Autodesk Inventor part; units mm, degrees
(part 2 of 2)
  line L990 (56.4, 473.8891) -> (43.8, 481.1637)
  line L991 (43.8, 481.1637) -> (43.8, 495.7129)
  line L992 (43.8, 495.7129) -> (56.4, 502.9876)
  line L993 (42.3, 527.4095) -> (54.9, 520.1349)
  line L994 (54.9, 520.1349) -> (54.9, 505.5856)
  line L995 (54.9, 505.5856) -> (42.3, 498.311)
  line L996 (42.3, 498.311) -> (29.7, 505.5856)
  line L997 (29.7, 505.5856) -> (29.7, 520.1349)
  line L998 (29.7, 520.1349) -> (42.3, 527.4095)
  line L999 (28.2, 551.8314) -> (40.8, 544.5568)
  line L1000 (40.8, 544.5568) -> (40.8, 530.0075)
  line L1001 (40.8, 530.0075) -> (28.2, 522.7329)
  line L1002 (28.2, 522.7329) -> (15.6, 530.0075)
  line L1003 (15.6, 530.0075) -> (15.6, 544.5568)
  line L1004 (15.6, 544.5568) -> (28.2, 551.8314)
  line L1005 (14.1, 576.2533) -> (26.7, 568.9787)
  line L1006 (26.7, 568.9787) -> (26.7, 554.4295)
  line L1007 (26.7, 554.4295) -> (14.1, 547.1549)
  line L1008 (14.1, 547.1549) -> (1.5, 554.4295)
  line L1009 (1.5, 554.4295) -> (1.5, 568.9787)
  line L1010 (1.5, 568.9787) -> (14.1, 576.2533)
  line L1011 (0, 600.6752) -> (12.6, 593.4006)
  line L1012 (12.6, 593.4006) -> (12.6, 578.8514)
  line L1013 (12.6, 578.8514) -> (0, 571.5768)
  line L1014 (0, 571.5768) -> (-12.6, 578.8514)
  line L1015 (-12.6, 578.8514) -> (-12.6, 593.4006)
  line L1016 (-12.6, 593.4006) -> (0, 600.6752)
  line L1017 (75, 218.063) -> (-75, 218.063)
  line L1018 (-75, 218.063) -> (-75, 368.063)
  line L1019 (-75, 368.063) -> (75, 368.063)
  line L1020 (75, 368.063) -> (75, 218.063)
  line L1021 (75, 218.063) -> (-75, 368.063) construction
  line L1022 (-75, 218.063) -> (75, 368.063) construction
  point P0 (-14.1, 24.4219)
  point P1 (-20.4, 35.3338)
  point P2 (-7.6023, 35.6763)
  point P3 (-28.2, 48.8438)
  point P4 (-34.5, 59.7558)
  point P5 (-21.7023, 60.0982)
  point P6 (-42.3, 73.2657)
  point P7 (-48.6, 84.1777)
  point P8 (-35.8023, 84.5201)
  point P9 (-56.4, 97.6877)
  point P10 (-62.7, 108.5996)
  point P11 (-49.9023, 108.942)
  point P12 (-70.5, 122.1096)
  point P13 (-76.8, 133.0215)
  point P14 (-64.0023, 133.364)
  point P15 (-84.6, 146.5315)
  point P16 (-90.9, 157.4434)
  point P17 (-78.1023, 157.7859)
  point P18 (-98.7, 170.9534)
  point P19 (-105, 181.8653)
  point P20 (-92.2023, 182.2078)
  point P21 (-112.8, 195.3753)
  point P22 (-119.1, 206.2873)
  point P23 (-106.3023, 206.6297)
  point P24 (-126.9, 219.7972)
  point P25 (-133.2, 230.7092)
  point P26 (-120.4023, 231.0516)
  point P27 (-141, 244.2192)
  point P28 (-147.3, 255.1311)
  point P29 (-134.5023, 255.4735)
  point P30 (-155.1, 268.6411)
  point P31 (-161.4, 279.553)
  point P32 (-148.6023, 279.8955)
  point P33 (-169.2, 293.063)
  point P34 (-175.5, 303.9749)
  point P35 (-162.7023, 304.3174)
  point P36 (14.1, 24.4219)
  point P37 (7.8, 35.3338)
  point P38 (20.5977, 35.6763)
  point P39 (0, 48.8438)
  point P40 (-6.3, 59.7558)
  point P41 (6.4977, 60.0982)
  point P42 (-14.1, 73.2657)
  point P43 (-20.4, 84.1777)
  point P44 (-7.6023, 84.5201)
  point P45 (-28.2, 97.6877)
  point P46 (-34.5, 108.5996)
  point P47 (-21.7023, 108.942)
  point P48 (-42.3, 122.1096)
  point P49 (-48.6, 133.0215)
  point P50 (-35.8023, 133.364)
  point P51 (-56.4, 146.5315)
  point P52 (-62.7, 157.4434)
  point P53 (-49.9023, 157.7859)
  point P54 (-70.5, 170.9534)
  point P55 (-76.8, 181.8653)
  point P56 (-64.0023, 182.2078)
  point P57 (-84.6, 195.3753)
  point P58 (-90.9, 206.2873)
  point P59 (-78.1023, 206.6297)
  point P60 (-98.7, 219.7972)
  point P61 (-105, 230.7092)
  point P62 (-92.2023, 231.0516)
  point P63 (-112.8, 244.2192)
  point P64 (-119.1, 255.1311)
  point P65 (-106.3023, 255.4735)
  point P66 (-126.9, 268.6411)
  point P67 (-133.2, 279.553)
  point P68 (-120.4023, 279.8955)
  point P69 (-141, 293.063)
  point P70 (-147.3, 303.9749)
  point P71 (-134.5023, 304.3174)
  point P72 (-155.1, 317.4849)
  point P73 (-161.4, 328.3968)
  point P74 (-148.6023, 328.7393)
  point P75 (28.2, 48.8438)
  point P76 (21.9, 59.7558)
  point P77 (34.6977, 60.0982)
  point P78 (14.1, 73.2657)
  point P79 (7.8, 84.1777)
  point P80 (20.5977, 84.5201)
  point P81 (0, 97.6877)
  point P82 (-6.3, 108.5996)
  point P83 (6.4977, 108.942)
  point P84 (-14.1, 122.1096)
  point P85 (-20.4, 133.0215)
  point P86 (-7.6023, 133.364)
  point P87 (-28.2, 146.5315)
  point P88 (-34.5, 157.4434)
  point P89 (-21.7023, 157.7859)
  point P90 (-42.3, 170.9534)
  point P91 (-48.6, 181.8653)
  point P92 (-35.8023, 182.2078)
  point P93 (-56.4, 195.3753)
  point P94 (-62.7, 206.2873)
  point P95 (-49.9023, 206.6297)
  point P96 (-70.5, 219.7972)
  point P97 (-76.8, 230.7092)
  point P98 (-64.0023, 231.0516)
  point P99 (-84.6, 244.2192)
  point P100 (-90.9, 255.1311)
  point P101 (-78.1023, 255.4735)
  point P102 (-98.7, 268.6411)
  point P103 (-105, 279.553)
  point P104 (-92.2023, 279.8955)
  point P105 (-112.8, 293.063)
  point P106 (-119.1, 303.9749)
  point P107 (-106.3023, 304.3174)
  point P108 (-126.9, 317.4849)
  point P109 (-133.2, 328.3968)
  point P110 (-120.4023, 328.7393)
  point P111 (-141, 341.9068)
  point P112 (-147.3, 352.8187)
  point P113 (-134.5023, 353.1612)
  point P114 (42.3, 73.2657)
  point P115 (36, 84.1777)
  point P116 (48.7977, 84.5201)
  point P117 (28.2, 97.6877)
  point P118 (21.9, 108.5996)
  point P119 (34.6977, 108.942)
  point P120 (14.1, 122.1096)
  point P121 (7.8, 133.0215)
  point P122 (20.5977, 133.364)
  point P123 (0, 146.5315)
  point P124 (-6.3, 157.4434)
  point P125 (6.4977, 157.7859)
  point P126 (-14.1, 170.9534)
  point P127 (-20.4, 181.8653)
  point P128 (-7.6023, 182.2078)
  point P129 (-28.2, 195.3753)
  point P130 (-34.5, 206.2873)
  point P131 (-21.7023, 206.6297)
  point P132 (-42.3, 219.7972)
  point P133 (-48.6, 230.7092)
  point P134 (-35.8023, 231.0516)
  point P135 (-56.4, 244.2192)
  point P136 (-62.7, 255.1311)
  point P137 (-49.9023, 255.4735)
  point P138 (-70.5, 268.6411)
  point P139 (-76.8, 279.553)
  point P140 (-64.0023, 279.8955)
  point P141 (-84.6, 293.063)
  point P142 (-90.9, 303.9749)
  point P143 (-78.1023, 304.3174)
  point P144 (-98.7, 317.4849)
  point P145 (-105, 328.3968)
  point P146 (-92.2023, 328.7393)
  point P147 (-112.8, 341.9068)
  point P148 (-119.1, 352.8187)
  point P149 (-106.3023, 353.1612)
  point P150 (-126.9, 366.3287)
  point P151 (-133.2, 377.2407)
  point P152 (-120.4023, 377.5831)
  point P153 (56.4, 97.6877)
  point P154 (50.1, 108.5996)
  point P155 (62.8977, 108.942)
  point P156 (42.3, 122.1096)
  point P157 (36, 133.0215)
  point P158 (48.7977, 133.364)
  point P159 (28.2, 146.5315)
  point P160 (21.9, 157.4434)
  point P161 (34.6977, 157.7859)
  point P162 (14.1, 170.9534)
  point P163 (7.8, 181.8653)
  point P164 (20.5977, 182.2078)
  point P165 (0, 195.3753)
  point P166 (-6.3, 206.2873)
  point P167 (6.4977, 206.6297)
  point P168 (-14.1, 219.7972)
  point P169 (-20.4, 230.7092)
  point P170 (-7.6023, 231.0516)
  point P171 (-28.2, 244.2192)
  point P172 (-34.5, 255.1311)
  point P173 (-21.7023, 255.4735)
  point P174 (-42.3, 268.6411)
  point P175 (-48.6, 279.553)
  point P176 (-35.8023, 279.8955)
  point P177 (-56.4, 293.063)
  point P178 (-62.7, 303.9749)
  point P179 (-49.9023, 304.3174)
  point P180 (-70.5, 317.4849)
  point P181 (-76.8, 328.3968)
  point P182 (-64.0023, 328.7393)
  point P183 (-84.6, 341.9068)
  point P184 (-90.9, 352.8187)
  point P185 (-78.1023, 353.1612)
  point P186 (-98.7, 366.3287)
  point P187 (-105, 377.2407)
  point P188 (-92.2023, 377.5831)
  point P189 (-112.8, 390.7507)
  point P190 (-119.1, 401.6626)
  point P191 (-106.3023, 402.005)
  point P192 (70.5, 122.1096)
  point P193 (64.2, 133.0215)
  point P194 (76.9977, 133.364)
  point P195 (56.4, 146.5315)
  point P196 (50.1, 157.4434)
  point P197 (62.8977, 157.7859)
  point P198 (42.3, 170.9534)
  point P199 (36, 181.8653)
  dimension "d0" = 14.5492
  dimension "d3" = 28.2
  dimension "d6" = 28.2
  dimension "d40" = 150
  dimension "d41" = 150
  constraints: 2046 end point, 171 midpoint, 3 perpendicular, 2 parallel, 1 coincident, 1 horizontal, 1 vertical, 2535 other
  measures "d0" distance of L0.start L0.end
  measures "d3" distance of L0.end L9.start
  measures "d6" distance of L0.end L81.start
  measures "d40" distance of L1018.end L1019.end
  measures "d41" distance of L1017.end L1018.end
extrude "Extrusion_HoneyComb" add sketch "Sketch1" along normal blind 3 contours L206 L1018 L209 L208 L207 L288 L287 L286 L285 L290 L293 L292 L291 L372 L371 L370 L369 L374 L377 L376 L375 L456 L455 L454 L1019 L529 L528 L527 L526 L601 L600 L599 L598 L673 L672 L671 L670 L745 L744 L743 L742 L817 L816 L815 L1020 L812 L811 L810 L729 L734 L733 L732 L731 L728 L727 L726 L645 L650 L649 L648 L647 L644 L643 L642 L561 L566 L565 L1017 L490 L489 L494 L493 L418 L417 L422 L421 L346 L345 L350 L349 L274 L273 L278 L277 L202 L201 | L201 L202 L1017 L1018 L206 | L1018 L207 L208 L209 | L277 L278 L273 L274 L1017 | L1018 L290 L285 L286 L287 L288 | L349 L350 L345 L346 L1017 | L1018 L291 L292 L293 | L421 L422 L417 L418 L1017 | L1018 L374 L369 L370 L371 L372 | L493 L494 L489 L490 L1017 | L1018 L375 L376 L377 | L565 L566 L561 L1020 L1017 | L1018 L1019 L454 L455 L456 | L642 L643 L644 L1020 | L1019 L526 L527 L528 L529 | L647 L648 L649 L650 L645 L1020 | L1019 L598 L599 L600 L601 | L726 L727 L728 L1020 | L1019 L670 L671 L672 L673 | L731 L732 L733 L734 L729 L1020 | L1019 L742 L743 L744 L745 | L810 L811 L812 L1020 | L1019 L1020 L815 L816 L817
sketch "Sketch2" plane through (0, 0, 0) normal (0, 0, -1) x (-1, 0, 0)
  line L0 (-75, 368.063) -> (-75, 218.063) projected
  line L1 (-75, 368.063) -> (-72, 368.063)
  line L2 (-72, 368.063) -> (-72, 330.563)
  line L3 (-72, 330.563) -> (-75, 330.563)
  line L4 (-75, 330.563) -> (-75, 368.063)
  line L5 (-75, 330.563) -> (-72, 330.563)
  line L6 (-72, 330.563) -> (-72, 293.063)
  line L7 (-72, 293.063) -> (-75, 293.063)
  line L8 (-75, 293.063) -> (-75, 330.563)
  line L9 (-75, 293.063) -> (-72, 293.063)
  line L10 (-72, 293.063) -> (-72, 255.563)
  line L11 (-72, 255.563) -> (-75, 255.563)
  line L12 (-75, 255.563) -> (-75, 293.063)
  line L13 (75, 218.063) -> (-75, 218.063) projected
  line L14 (-75, 255.563) -> (-72, 255.563)
  line L15 (-72, 255.563) -> (-72, 218.063)
  line L16 (-72, 218.063) -> (-75, 218.063)
  line L17 (-75, 218.063) -> (-75, 255.563)
  line L18 (-75, 218.063) -> (-37.5, 218.063)
  line L19 (-37.5, 218.063) -> (-37.5, 221.063)
  line L20 (-37.5, 221.063) -> (-75, 221.063)
  line L21 (-75, 221.063) -> (-75, 218.063)
  line L22 (-37.5, 218.063) -> (0, 218.063)
  line L23 (0, 218.063) -> (0, 221.063)
  line L24 (0, 221.063) -> (-37.5, 221.063)
  line L25 (-37.5, 221.063) -> (-37.5, 218.063)
  line L26 (0, 218.063) -> (37.5, 218.063)
  line L27 (37.5, 218.063) -> (37.5, 221.063)
  line L28 (37.5, 221.063) -> (0, 221.063)
  line L29 (0, 221.063) -> (0, 218.063)
  line L30 (75, 368.063) -> (75, 218.063) projected
  line L31 (37.5, 218.063) -> (75, 218.063)
  line L32 (75, 218.063) -> (75, 221.063)
  line L33 (75, 221.063) -> (37.5, 221.063)
  line L34 (37.5, 221.063) -> (37.5, 218.063)
  line L35 (75, 218.063) -> (72, 218.063)
  line L36 (72, 218.063) -> (72, 255.563)
  line L37 (72, 255.563) -> (75, 255.563)
  line L38 (75, 255.563) -> (75, 218.063)
  line L39 (75, 255.563) -> (72, 255.563)
  line L40 (72, 255.563) -> (72, 293.063)
  line L41 (72, 293.063) -> (75, 293.063)
  line L42 (75, 293.063) -> (75, 255.563)
  line L43 (75, 293.063) -> (72, 293.063)
  line L44 (72, 293.063) -> (72, 330.563)
  line L45 (72, 330.563) -> (75, 330.563)
  line L46 (75, 330.563) -> (75, 293.063)
  line L47 (-75, 368.063) -> (75, 368.063) projected
  line L48 (75, 330.563) -> (72, 330.563)
  line L49 (72, 330.563) -> (72, 368.063)
  line L50 (72, 368.063) -> (75, 368.063)
  line L51 (75, 368.063) -> (75, 330.563)
  line L52 (-75, 368.063) -> (-37.5, 368.063)
  line L53 (-37.5, 368.063) -> (-37.5, 365.063)
  line L54 (-37.5, 365.063) -> (-75, 365.063)
  line L55 (-75, 365.063) -> (-75, 368.063)
  line L56 (-37.5, 368.063) -> (0, 368.063)
  line L57 (0, 368.063) -> (0, 365.063)
  line L58 (0, 365.063) -> (-37.5, 365.063)
  line L59 (-37.5, 365.063) -> (-37.5, 368.063)
  line L60 (0, 368.063) -> (37.5, 368.063)
  line L61 (37.5, 368.063) -> (37.5, 365.063)
  line L62 (37.5, 365.063) -> (0, 365.063)
  line L63 (0, 365.063) -> (0, 368.063)
  line L64 (37.5, 368.063) -> (75, 368.063)
  line L65 (75, 368.063) -> (75, 365.063)
  line L66 (75, 365.063) -> (37.5, 365.063)
  line L67 (37.5, 365.063) -> (37.5, 368.063)
  point P0 (0, 0)
  dimension "d44" = 3
  dimension "d45" = 37.5
  dimension "d46" = 3
  dimension "d47" = 37.5
  dimension "d48" = 3
  dimension "d49" = 37.5
  dimension "d50" = 3
  dimension "d51" = 37.5
  dimension "d52" = 3
  dimension "d53" = 37.5
  dimension "d54" = 3
  dimension "d55" = 37.5
  dimension "d56" = 3
  dimension "d57" = 3
  dimension "d58" = 37.5
  dimension "d59" = 3
  dimension "d60" = 37.5
  dimension "d61" = 37.5
  dimension "d62" = 37.5
  dimension "d63" = 3
  dimension "d64" = 37.5
  dimension "d65" = 3
  dimension "d66" = 37.5
  dimension "d67" = 3
  constraints: 128 end point, 32 parallel, 16 horizontal, 16 perpendicular, 8 point on line
  measures "d44" distance of L2.end L3.end
  measures "d45" distance of L1.end L2.end
  measures "d46" distance of L6.end L7.end
  measures "d47" distance of L5.end L6.end
  measures "d48" distance of L10.end L11.end
  measures "d49" distance of L9.end L10.end
  measures "d50" distance of L15.end L16.end
  measures "d51" distance of L20.end L19.end
  measures "d52" distance of L19.end L18.end
  measures "d53" distance of L24.end L23.end
  measures "d54" distance of L23.end L22.end
  measures "d55" distance of L28.end L27.end
  measures "d56" distance of L27.end L26.end
  measures "d57" distance of L36.end L37.end
  measures "d58" distance of L35.end L36.end
  measures "d59" distance of L40.end L41.end
  measures "d60" distance of L39.end L40.end
  measures "d61" distance of L43.end L44.end
  measures "d62" distance of L53.end L54.end
  measures "d63" distance of L52.end L53.end
  measures "d64" distance of L57.end L58.end
  measures "d65" distance of L56.end L57.end
  measures "d66" distance of L61.end L62.end
  measures "d67" distance of L60.end L61.end
extrude "Extrusion_Overlay" cut sketch "Sketch2" against normal blind 62.0875 contours L1 L2 L54 L0 | L47 L53 L54 L2 | L3 L6 L7 L0 | L47 L61 L62 L57 | L11 L15 L20 L0 | L20 L15 L13 L0 | L47 L30 L66 L49 | L66 L30 L45 L49 | L24 L23 L13 L19 | L41 L30 L37 L40 | L33 L36 L13 L27 | L33 L30 L13 L36
body "Solid2"
